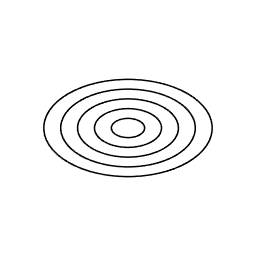
Bed Check v2 (Autodesk Fusion 360 design; units mm, degrees)
Autodesk Fusion 360 part; units mm, degrees
sketch "Sketch1" plane through (0, 0, 0) normal (0, 0, 1) x (1, 0, 0)
  circle A0 centre (94, 87) radius 75
  circle A1 centre (94, 87) radius 45
  circle A2 centre (94, 87) radius 15
  circle A3 centre (94, 87) radius 60
  circle A4 centre (94, 87) radius 30
  circle A5 centre (94, 87) radius 74.52
  circle A6 centre (94, 87) radius 59.52
  circle A7 centre (94, 87) radius 44.52
  circle A8 centre (94, 87) radius 29.52
  circle A9 centre (94, 87) radius 14.52
  dimension "d1" = 150
  dimension "d2" = -30
  dimension "d3" = -60
  dimension "d4" = -15
  dimension "d5" = -45
  dimension "d6" = -0.48
  dimension "d7" = -15.48
  dimension "d8" = -30.48
  dimension "d9" = -45.48
  dimension "d10" = -60.48
  measures "d1" diameter of A0
extrude "Extrude1" add sketch "Sketch1" along normal blind 0.2 makes body 1 at (81.8799, 130.055, 0) makes body 2 at (153.6166, 89.9808, 0) makes body 3 at (103.4736, 58.7822, 0) makes body 4 at (168.5608, 90.7261, 0) makes body 5 at (82.6556, 96.5095, 0)
